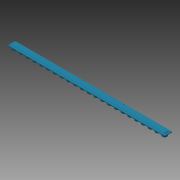
# Autodesk Inventor part: 载板滚柱挡板
Saved by Autodesk Inventor 2015 (Build 190159000, 159)
## iProperties
Created: 2017-05-05
Part Number: 载板滚柱挡板
Material: 常规
Document SubType Name: Modeling
Designer: Administrator
Density: 1 g/cm^3
Appearance: 青绿色
Author: Administrator
Autodesk Inventor part; units mm, degrees
ref_plane "YZ Plane" through (0, 0, 0) normal (1, 0, 0) x (0, 1, 0)
ref_plane "XZ Plane" through (0, 0, 0) normal (0, 1, 0) x (-1, 0, 0)
ref_plane "XY Plane" through (0, 0, 0) normal (0, 0, 1) x (1, 0, 0)
sketch "草图1" plane through (0, 0, 0) normal (0, 0, 1) x (1, 0, 0)
  line L0 (0, 0) -> (1155, 0)
  line L1 (1155, 0) -> (1155, -55)
  line L2 (1155, -55) -> (0, -55)
  line L3 (0, -55) -> (0, 0)
  dimension "d0" = 1155
  dimension "d1" = 55
  constraints: 8 end point, 2 parallel, 1 coincident, 1 horizontal, 1 perpendicular
  measures "d0" distance of L0.start L0.end
  measures "d1" distance of L0.end L1.end
extrude "拉伸1" add sketch "草图1" along normal blind 10
sketch "草图2" plane through (0, -55, 0) normal (-1, 0, 0) x (0, 0, 1)
  line L0 (0, 55) -> (10, 55) projected
  line L1 (5, 55) -> (5, 45)
  line L2 (5, 45) -> (10, 40)
  line L3 (10, 55) -> (10, 0) projected
  line L4 (0, 0) -> (10, 0) projected
  line L5 (5, 0) -> (5, 10)
  line L6 (5, 10) -> (10, 15)
  dimension "d4" = 10
  dimension "d5" = 10
  dimension "d6" = 5
  dimension "d7" = 5
  constraints: 8 end point, 3 point on line, 2 midpoint, 1 vertical
  measures "d4" distance of L1.start L1.end
  measures "d5" distance of L5.start L5.end
  measures "d6" horizontal distance of L5.end L6.end
  measures "d7" horizontal distance of L1.end L2.end
extrude "拉伸2" cut sketch "草图2" against normal blind 1155
sketch "草图3" plane through (0, -55, 0) normal (0, -1, 0) x (1, 0, 0)
  line L0 (0, 5) -> (10, 5)
  line L1 (0, 5) -> (1155, 5) projected
  line L2 (10, 5) -> (15, 10)
  line L3 (1155, 10) -> (0, 10) projected
  line L4 (1155, 5) -> (1145, 5)
  line L5 (1145, 5) -> (1140, 10)
  line L6 (0, 5) -> (0, 10)
  line L7 (15, 10) -> (0, 10)
  line L8 (1140, 10) -> (1155, 10)
  line L9 (1155, 5) -> (1155, 10)
  line L10 (1155, 5) -> (1155, 10) projected
  point P0 (0, 0)
  dimension "d10" = 10
  dimension "d11" = 5
  dimension "d12" = 10
  dimension "d13" = 5
  dimension "d14" = 135
  constraints: 16 end point, 3 point on line, 2 perpendicular, 1 collinear
  measures "d10" distance of L0.start L0.end
  measures "d11" horizontal distance of L2.end L0.end
  measures "d12" distance of L1.end L4.end
  measures "d13" horizontal distance of L5.end L4.end
  measures "d14" angle of L1 L5
extrude "拉伸3" cut sketch "草图3" against normal blind 55 contours L6 L3 L2 L0 | L5 L3 L9 L1
sketch "草图4" plane through (0, 0, 0) normal (0, 0, -1) x (-1, 0, 0)
  circle A0 centre (-27.5, -27.5) radius 17.5
  circle A1 centre (-27.5, -27.5) radius 13.75
  line L0 (-10, -10) -> (-1145, -10) projected
  point P0 (0, 0)
  dimension "d17" = 27.5
  dimension "d18" = 27.5
  dimension "d19" = 3.75
  constraints: 2 centre point, 1 coincident, 1 tangent
  measures "d17" horizontal distance of point (0, 0) A1.centre
  measures "d18" horizontal distance of point (0, 0) A0.centre
  measures "d19" radial gap between concentric circles of A0 A1
extrude "拉伸4" add sketch "草图4" along normal blind 20
sketch "草图5" plane through (27.5, -27.5, -20) normal (0, 0, -1) x (-1, 0, 0)
  circle A0 centre (0, 0) radius 17.5
  circle A1 centre (0, 0) radius 13.75
  circle A2 centre (0, 0) radius 13.75 projected
  circle A3 centre (0, 0) radius 17.5 projected
  circle A4 centre (0, 0) radius 17.5 projected
  line L0 (1.5, -17.4356) -> (1.5, 17.4356)
  line L1 (-1.5, -17.4356) -> (-1.5, 17.4356)
  line L2 (17.4356, 1.5) -> (-17.4356, 1.5)
  line L3 (-17.4356, -1.5) -> (17.4356, -1.5)
  line L4 (17.5, 17.5) -> (-1117.5, 17.5) projected
  point P0 (27.5, 27.5)
  dimension "d22" = 1.5
  dimension "d23" = 1.5
  dimension "d24" = 1.5
  dimension "d25" = 1.5
  constraints: 8 end point, 4 perpendicular, 2 centre point, 2 coincident, 1 concentric, 19 other
  measures "d22" distance from line of A0.centre L3
  measures "d23" distance from line of L2 A0.centre
  measures "d24" distance from line of A0.centre L0
  measures "d25" distance from line of A0.centre L1
extrude "拉伸5" cut sketch "草图5" against normal blind 10 contours A0 L3 A1 L2 | L0 A1 L1 A0 | A1 L3 L0 L2 | A0 L1 A1 L0 | L0 L2 L1 A1 | L0 L3 L1 L2 | A1 L1 L3 L0 | L1 L3 A1 L2 | A0 L2 A1 L3
pattern_linear "矩形阵列1" count 23 spacing 50 along (1, 0, 0) of "拉伸5", "拉伸4"
sketch "草图6" plane through (0, -55, 5) normal (0, 0, 1) x (1, 0, 0)
  circle A0 centre (5, 50) radius 2
  circle A1 centre (5, 5) radius 2
  line L0 (0, 55) -> (1155, 55) projected
  line L1 (0, 0) -> (0, 55) projected
  line L2 (1155, 0) -> (0, 0) projected
  dimension "d31" = 4
  dimension "d32" = 4
  dimension "d33" = 5
  dimension "d34" = 5
  dimension "d35" = 5
  dimension "d36" = 5
  constraints: 2 centre point
  measures "d31" diameter of A0
  measures "d32" diameter of A1
  measures "d33" distance from line of L0 A0.centre
  measures "d34" distance from line of L1 A0.centre
  measures "d35" distance from line of L1 A1.centre
  measures "d36" distance from line of L2 A1.centre
extrude "拉伸6" cut sketch "草图6" against normal blind 5
pattern_linear "矩形阵列3" count 2 spacing 197.5 along (1, 0, 0) of "拉伸6"
pattern_linear "矩形阵列4" count 6 spacing 150 along (1, 0, 0) of "矩形阵列3"
pattern_linear "矩形阵列5" count 2 spacing 1145 along (1, 0, 0) of "拉伸6"
